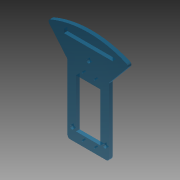
# Autodesk Inventor part: bracket_camera_top
Saved by Autodesk Inventor 2015 SP2 (Build 190223200, 223)
## iProperties
Created: 2015-10-08
Part Number: bracket_camera_top
Material: Generic
Document SubType Name: Modeling
Designer: styku
Density: 1 g/cm^3
Appearance: Clear
Author: styku
Autodesk Inventor part; units mm, degrees
ref_plane "YZ Plane" through (0, 0, 0) normal (1, 0, 0) x (0, 1, 0)
ref_plane "XZ Plane" through (0, 0, 0) normal (0, 1, 0) x (-1, 0, 0)
ref_plane "XY Plane" through (0, 0, 0) normal (0, 0, 1) x (1, 0, 0)
sketch "Sketch1" plane through (0, 0, 0) normal (0, 1, 0) x (-1, 0, 0)
  line L0 (46, 0) -> (-35, 0) construction
  line L1 (0, 54.3949) -> (0, -60) construction
  line L2 (10, 20) -> (-10, 20)
  line L3 (-10, 20) -> (-10, -20)
  line L4 (-10, -20) -> (10, -20)
  line L5 (10, -20) -> (10, 20)
  line L6 (17, -28) -> (17, 28)
  circle A0 centre (5, 24.25) radius 0.5
  circle A1 centre (-5, 24.25) radius 0.5
  line L7 (14.6784, 24.25) -> (-18, 24.25) construction
  circle A2 centre (5, -24.25) radius 0.5
  circle A3 centre (-5, -24.25) radius 0.5
  circle A4 centre (13.5, -18.75) radius 1.5
  line L8 (-17, 28) -> (-17, -28)
  line L9 (17, -28) -> (-17, -28)
  line L10 (17, 28) -> (33.782, 48)
  line L11 (17, 28) -> (43.1081, 28) construction
  line L12 (-17, 28) -> (-33.782, 48)
  arc A5 (33.782, 48) -> (-33.782, 48) centre (0, -24.5174) ccw
  line L13 (20, 48) -> (-20, 48)
  line L14 (-20, 48) -> (-20, 45)
  line L15 (-20, 45) -> (20, 45)
  line L16 (20, 45) -> (20, 48)
  circle A6 centre (0, 35) radius 1.5
  circle A7 centre (-13.5, -18.75) radius 1.5
  point P0 (0, 0)
  dimension "d0" = 40
  dimension "d1" = 20
  dimension "d2" = 7
  dimension "d6" = 20
  dimension "d7" = 10
  dimension "d11" = 1
  dimension "d12" = 1
  dimension "d13" = 5
  dimension "d14" = 5
  dimension "d15" = 4.25
  dimension "d16" = 3
  dimension "d29" = 3.5
  dimension "d34" = 8
  dimension "d35" = 50
  dimension "d36" = 20
  dimension "d37" = 56
  dimension "d38" = 80
  dimension "d39" = 40
  dimension "d41" = 3
  dimension "d42" = 25
  dimension "d43" = 9.25
  dimension "d44" = 3
  dimension "d45" = 10
  constraints: 34 end point, 8 centre point, 5 horizontal, 5 perpendicular, 4 symmetric about line, 4 vertical, 3 point on line, 2 equal length, 2 parallel, 2 point on circle, 5 other
  measures "d0" distance between parallel lines of L4 L2
  measures "d1" distance between parallel lines of L3 L5
  measures "d2" distance between parallel lines of L5 L6
  measures "d6" distance between parallel lines of L0 L2
  measures "d7" distance between parallel lines of L1 L5
  measures "d11" diameter of A1
  measures "d12" diameter of A0
  measures "d13" distance from line of A0.centre L5
  measures "d14" distance from line of L3 A1.centre
  measures "d15" distance between parallel lines of L2 L7
  measures "d16" diameter of A4
  measures "d29" distance from line of L5 A4.centre
  measures "d34" distance between parallel lines of L9 L4
  measures "d35" angle of L11 L10
  measures "d36" vertical distance of L8.start L12.end
  measures "d37" distance of L8.start L8.end
  measures "d38" radius of A5
  measures "d39" distance of L13.start L13.end
  measures "d41" distance of L13.end L14.end
  measures "d42" distance between parallel lines of L2 L15
  measures "d43" distance from line of L9 A4.centre
  measures "d44" diameter of A6
  measures "d45" distance from line of L15 A6.centre
extrude "Extrusion2" add sketch "Sketch1" along normal blind 3
fillet "Fillet2" radius 2 6 edges at (33.782, 1.5, 48) (-33.782, 1.5, 48) (17, 1.5, 28) (-17, 1.5, 28) (-17, 1.5, -28) (17, 1.5, -28)
body "Solid2"
